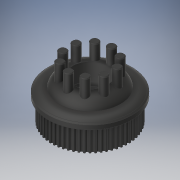
# Autodesk Inventor part: Orangatang Kegel Flat Face Adapter_2
Saved by Autodesk Inventor 2019.2 (Build 232265000, 265)
## iProperties
Created: 2018-11-27
Part Number: Orangatang Kegel Flat Face Adapter_2
Material: Aluminum 6061-AHC
Document SubType Name: Modeling
Designer: Petar
Density: 2.7 g/cm^3
Appearance: Smooth - Black
Author: Petar
Autodesk Inventor part; units mm, degrees
ref_plane "YZ Plane" through (0, 0, 0) normal (1, 0, 0) x (0, 1, 0)
ref_plane "XZ Plane" through (0, 0, 0) normal (0, 1, 0) x (-1, 0, 0)
ref_plane "XY Plane" through (0, 0, 0) normal (0, 0, 1) x (1, 0, 0)
derived "gates_P60-3M-09AL.ipt"
sketch "Sketch2_1" plane through (-27.813, -17.4625, 4.73202) normal (0, -1, 0) x (0.7504539, 0, 0.6609228)
  arc A0 (-0.667833, -0.547543) -> (0.667833, -0.547543) centre (0, 0) ccw
  arc A1 (-0.667833, -0.547543) -> (-1.061506, -0.54856) centre (-0.864255, -0.708586) ccw
  arc A2 (-1.061506, -0.54856) -> (-1.467465, -1.060953) centre (20.892519, -18.359372) ccw
  arc A3 (-1.467465, -1.060953) -> (-1.389566, -1.459114) centre (-1.254213, -1.225932) ccw
  arc A4 (-1.083217, -2.759174) -> (-1.389566, -1.459114) centre (-1.850942, -2.253958) ccw
  arc A5 (-2.411566, -2.898789) -> (-1.083217, -2.759174) centre (-1.804626, -2.284437) ccw
  arc A6 (-2.411566, -2.898789) -> (-2.802976, -2.94095) centre (-2.590078, -3.079481) ccw
  arc A7 (-2.802976, -2.94095) -> (-3.153152, -3.49297) centre (20.892519, -18.359372) ccw
  arc A8 (-3.153152, -3.49297) -> (-3.03406, -3.880808) centre (-2.923823, -3.634754) ccw
  arc A9 (-2.593496, -5.141723) -> (-3.03406, -3.880808) centre (-3.409825, -4.719524) ccw
  arc A10 (-3.899975, -5.419424) -> (-2.593496, -5.141723) centre (-3.360576, -4.744995) ccw
  arc A11 (-3.899975, -5.419424) -> (-4.284833, -5.502268) centre (-4.058622, -5.617785) ccw
  arc A12 (-4.284833, -5.502268) -> (-4.575389, -6.087867) centre (20.892519, -18.359372) ccw
  arc A13 (-4.575389, -6.087867) -> (-4.41641, -6.461132) centre (-4.332496, -6.204903) ccw
  arc A14 (-3.846458, -7.669088) -> (-4.41641, -6.461132) centre (-4.702447, -7.334531) ccw
  arc A15 (-5.116752, -8.081832) -> (-3.846458, -7.669088) centre (-4.650805, -7.354715) ccw
  arc A16 (-5.116752, -8.081832) -> (-5.490843, -8.20445) centre (-5.253795, -8.295689) ccw
  arc A17 (-5.490843, -8.20445) -> (-5.718595, -8.817212) centre (20.892519, -18.359372) ccw
  arc A18 (-5.718595, -8.817212) -> (-5.52147, -9.171815) centre (-5.464799, -8.908218) ccw
  arc A19 (-4.828374, -10.313578) -> (-5.52147, -9.171815) centre (-5.714644, -10.070329) ccw
  arc A20 (-6.048566, -10.856842) -> (-4.828374, -10.313578) centre (-5.661176, -10.085004) ccw
  arc A21 (-6.048566, -10.856842) -> (-6.40779, -11.017892) centre (-6.162504, -11.083853) ccw
  arc A22 (-6.40779, -11.017892) -> (-6.570244, -11.651104) centre (20.892519, -18.359372) ccw
  arc A23 (-6.570244, -11.651104) -> (-6.337133, -11.983159) centre (-6.308325, -11.715083) ccw
  arc A24 (-5.528487, -13.046219) -> (-6.337133, -11.983159) centre (-6.435328, -12.896943) ccw
  arc A25 (-6.685208, -13.714052) -> (-5.528487, -13.046219) centre (-6.380619, -12.905949) ccw
  arc A26 (-6.685208, -13.714052) -> (-7.02563, -13.911769) centre (-6.774793, -13.951729) ccw
  arc A27 (-7.02563, -13.911769) -> (-7.121005, -14.558493) centre (20.892519, -18.359372) ccw
  arc A28 (-7.121005, -14.558493) -> (-6.854462, -14.864362) centre (-6.853833, -14.594743) ccw
  arc A29 (-5.939126, -15.837072) -> (-6.854462, -14.864362) centre (-6.856603, -15.783405) ccw
  arc A30 (-7.019703, -16.622157) -> (-5.939126, -15.837072) centre (-6.801252, -15.786643) ccw
  arc A31 (-7.019703, -16.622157) -> (-7.337593, -16.854375) centre (-7.083953, -16.867897) ccw
  arc A32 (-7.337593, -16.854375) -> (-7.364844, -17.507526) centre (20.892519, -18.359372) ccw
  arc A33 (-7.364844, -17.507526) -> (-7.067789, -17.783857) centre (-7.095347, -17.51565) ccw
  arc A34 (-6.055792, -18.65556) -> (-7.067789, -17.783857) centre (-6.973852, -18.698089) ccw
  arc A35 (-7.048385, -19.549295) -> (-6.055792, -18.65556) centre (-6.918466, -18.695524) ccw
  arc A36 (-7.048385, -19.549295) -> (-7.34026, -19.813469) centre (-7.086596, -19.800405) ccw
  arc A37 (-7.34026, -19.813469) -> (-7.29909, -20.465891) centre (20.892519, -18.359372) ccw
  arc A38 (-7.29909, -20.465891) -> (-6.974777, -20.709658) centre (-7.03022, -20.4458) ccw
  arc A39 (-5.877206, -21.470803) -> (-6.974777, -20.709658) centre (-6.785792, -21.609063) ccw
  arc A40 (-6.770941, -22.463397) -> (-5.877206, -21.470803) centre (-6.730978, -21.600722) ccw
  arc A41 (-6.770941, -22.463397) -> (-7.033604, -22.756633) centre (-6.782695, -22.717124) ccw
  arc A42 (-7.033604, -22.756633) -> (-6.924462, -23.401177) centre (20.892519, -18.359372) ccw
  arc A43 (-6.924462, -23.401177) -> (-6.576445, -23.609709) centre (-6.659165, -23.353092) ccw
  arc A44 (-5.405325, -24.251957) -> (-6.576445, -23.609709) centre (-6.294482, -24.484432) ccw
  arc A45 (-6.19041, -25.332533) -> (-5.405325, -24.251957) centre (-6.24084, -24.470407) ccw
  arc A46 (-6.19041, -25.332533) -> (-6.420982, -25.651619) centre (-6.175578, -25.5861) ccw
  arc A47 (-6.420982, -25.651619) -> (-6.245066, -26.281223) centre (20.892519, -18.359372) ccw
  arc A48 (-6.245066, -26.281223) -> (-5.877158, -26.452235) centre (-5.986248, -26.205671) ccw
  arc A49 (-4.64532, -26.96855) -> (-5.877158, -26.452235) centre (-5.505306, -27.292694) ccw
  arc A50 (-5.313153, -28.12527) -> (-4.64532, -26.96855) centre (-5.453423, -27.273138) ccw
  arc A51 (-5.313153, -28.12527) -> (-5.509109, -28.466709) centre (-5.271898, -28.375898) ccw
  arc A52 (-5.509109, -28.466709) -> (-5.268344, -29.074477) centre (20.892519, -18.359372) ccw
  arc A53 (-5.268344, -29.074477) -> (-4.884576, -29.206095) centre (-5.018842, -28.972284) ccw
  arc A54 (-3.605517, -29.590819) -> (-4.884576, -29.206095) centre (-4.426909, -30.00308) ccw
  arc A55 (-4.148782, -30.811011) -> (-3.605517, -29.590819) centre (-4.377355, -29.978209) ccw
  arc A56 (-4.148782, -30.811011) -> (-4.307974, -31.171062) centre (-4.081554, -31.055952) ccw
  arc A57 (-4.307974, -31.171062) -> (-4.004999, -31.750333) centre (20.892519, -18.359372) ccw
  arc A58 (-4.004999, -31.750333) -> (-3.609575, -31.841116) centre (-3.767545, -31.62262) ccw
  arc A59 (-2.297309, -32.090034) -> (-3.609575, -31.841116) centre (-3.071108, -32.585895) ccw
  arc A60 (-2.710052, -33.360328) -> (-2.297309, -32.090034) centre (-3.024425, -32.555981) ccw
  arc A61 (-2.710052, -33.360328) -> (-2.830737, -33.735047) centre (-2.61759, -33.596901) ccw
  arc A62 (-2.830737, -33.735047) -> (-2.468871, -34.279475) centre (20.892519, -18.359372) ccw
  arc A63 (-2.468871, -34.279475) -> (-2.066125, -34.328427) centre (-2.246068, -34.127641) ccw
  arc A64 (-0.735027, -34.438813) -> (-2.066125, -34.328427) centre (-1.452756, -35.012842) ccw
  arc A65 (-1.012728, -35.745291) -> (-0.735027, -34.438813) centre (-1.409456, -34.978211) ccw
  arc A66 (-1.012728, -35.745291) -> (-1.093582, -36.130573) centre (-0.896043, -35.970903) ccw
  arc A67 (-1.093582, -36.130573) -> (-0.676791, -36.634193) centre (20.892519, -18.359372) ccw
  arc A68 (-0.676791, -36.634193) -> (-0.271134, -36.640779) centre (-0.471079, -36.459902) ccw
  arc A69 (1.06421, -36.611422) -> (-0.271134, -36.640779) centre (0.410415, -37.25733) ccw
  arc A70 (0.924595, -37.939771) -> (1.06421, -36.611422) centre (0.449858, -37.218363) ccw
  arc A71 (0.924595, -37.939771) -> (0.884456, -38.331394) centre (1.064223, -38.15195) ccw
  arc A72 (0.884456, -38.331394) -> (1.351607, -38.788689) centre (20.892519, -18.359372) ccw
  arc A73 (1.351607, -38.788689) -> (1.75573, -38.752836) centre (1.537973, -38.593849) ccw
  arc A74 (3.08069, -38.584058) -> (1.75573, -38.752836) centre (2.497993, -39.294768) ccw
  arc A75 (3.08069, -39.919724) -> (3.08069, -38.584058) centre (2.533146, -39.251891) ccw
  arc A76 (3.08069, -39.919724) -> (3.081707, -40.313397) centre (3.241732, -40.116146) ccw
  arc A77 (3.081707, -40.313397) -> (3.594099, -40.719356) centre (20.892519, -18.359372) ccw
  arc A78 (3.594099, -40.719356) -> (3.992261, -40.641457) centre (3.759078, -40.506104) ccw
  arc A79 (5.29232, -40.335108) -> (3.992261, -40.641457) centre (4.787105, -41.102833) ccw
  arc A80 (5.431935, -41.663458) -> (5.29232, -40.335108) centre (4.817584, -41.056517) ccw
  arc A81 (5.431935, -41.663458) -> (5.474097, -42.054867) centre (5.612627, -41.84197) ccw
  arc A82 (5.474097, -42.054867) -> (6.026116, -42.405043) centre (20.892519, -18.359372) ccw
  arc A83 (6.026116, -42.405043) -> (6.413954, -42.285952) centre (6.167901, -42.175714) ccw
  arc A84 (7.67487, -41.845388) -> (6.413954, -42.285952) centre (7.252671, -42.661716) ccw
  arc A85 (7.95257, -43.151866) -> (7.67487, -41.845388) centre (7.278142, -42.612468) ccw
  arc A86 (7.95257, -43.151866) -> (8.035414, -43.536725) centre (8.150932, -43.310513) ccw
  arc A87 (8.035414, -43.536725) -> (8.621013, -43.827281) centre (20.892519, -18.359372) ccw
  arc A88 (8.621013, -43.827281) -> (8.994278, -43.668301) centre (8.738049, -43.584387) ccw
  arc A89 (10.202235, -43.098349) -> (8.994278, -43.668301) centre (9.867678, -43.954338) ccw
  arc A90 (10.614978, -44.368643) -> (10.202235, -43.098349) centre (9.887862, -43.902697) ccw
  arc A91 (10.614978, -44.368643) -> (10.737597, -44.742734) centre (10.828836, -44.505687) ccw
  arc A92 (10.737597, -44.742734) -> (11.350359, -44.970486) centre (20.892519, -18.359372) ccw
  arc A93 (11.350359, -44.970486) -> (11.704961, -44.773361) centre (11.441365, -44.71669) ccw
  arc A94 (12.846724, -44.080266) -> (11.704961, -44.773361) centre (12.603476, -44.966536) ccw
  arc A95 (13.389989, -45.300457) -> (12.846724, -44.080266) centre (12.618151, -44.913068) ccw
  arc A96 (13.389989, -45.300457) -> (13.551039, -45.659681) centre (13.617, -45.414396) ccw
  arc A97 (13.551039, -45.659681) -> (14.184251, -45.822135) centre (20.892519, -18.359372) ccw
  arc A98 (14.184251, -45.822135) -> (14.516305, -45.589024) centre (14.248229, -45.560216) ccw
  arc A99 (15.579365, -44.780378) -> (14.516305, -45.589024) centre (15.43009, -45.68722) ccw
  arc A100 (16.247199, -45.937099) -> (15.579365, -44.780378) centre (15.439095, -45.632511) ccw
  arc A101 (16.247199, -45.937099) -> (16.444915, -46.277521) centre (16.484876, -46.026684) ccw
  arc A102 (16.444915, -46.277521) -> (17.09164, -46.372896) centre (20.892519, -18.359372) ccw
  arc A103 (17.09164, -46.372896) -> (17.397509, -46.106353) centre (17.12789, -46.105725) ccw
  arc A104 (18.370219, -45.191017) -> (17.397509, -46.106353) centre (18.316551, -46.108494) ccw
  arc A105 (19.155304, -46.271594) -> (18.370219, -45.191017) centre (18.319789, -46.053144) ccw
  arc A106 (19.155304, -46.271594) -> (19.387521, -46.589484) centre (19.401043, -46.335844) ccw
  arc A107 (19.387521, -46.589484) -> (20.040672, -46.616735) centre (20.892519, -18.359372) ccw
  arc A108 (20.040672, -46.616735) -> (20.317004, -46.31968) centre (20.048796, -46.347238) ccw
  arc A109 (21.188707, -45.307683) -> (20.317004, -46.31968) centre (21.231236, -46.225744) ccw
  arc A110 (22.082442, -46.300276) -> (21.188707, -45.307683) centre (21.22867, -46.170358) ccw
  arc A111 (22.082442, -46.300276) -> (22.346616, -46.592151) centre (22.333551, -46.338488) ccw
  arc A112 (22.346616, -46.592151) -> (22.999037, -46.550981) centre (20.892519, -18.359372) ccw
  arc A113 (22.999037, -46.550981) -> (23.242805, -46.226668) centre (22.978947, -46.282111) ccw
  arc A114 (24.00395, -45.129097) -> (23.242805, -46.226668) centre (24.142209, -46.037683) ccw
  arc A115 (24.996543, -46.022832) -> (24.00395, -45.129097) centre (24.133868, -45.982869) ccw
  arc A116 (24.996543, -46.022832) -> (25.289779, -46.285495) centre (25.250271, -46.034586) ccw
  arc A117 (25.289779, -46.285495) -> (25.934323, -46.176353) centre (20.892519, -18.359372) ccw
  arc A118 (25.934323, -46.176353) -> (26.142855, -45.828337) centre (25.886238, -45.911056) ccw
  arc A119 (26.785103, -44.657217) -> (26.142855, -45.828337) centre (27.017578, -45.546373) ccw
  arc A120 (27.86568, -45.442302) -> (26.785103, -44.657217) centre (27.003553, -45.492731) ccw
  arc A121 (27.86568, -45.442302) -> (28.184765, -45.672874) centre (28.119246, -45.427469) ccw
  arc A122 (28.184765, -45.672874) -> (28.81437, -45.496957) centre (20.892519, -18.359372) ccw
  arc A123 (28.81437, -45.496957) -> (28.985382, -45.129049) centre (28.738817, -45.238139) ccw
  arc A124 (29.501696, -43.897212) -> (28.985382, -45.129049) centre (29.82584, -44.757197) ccw
  arc A125 (30.658417, -44.565045) -> (29.501696, -43.897212) centre (29.806285, -44.705315) ccw
  arc A126 (30.658417, -44.565045) -> (30.999856, -44.761) centre (30.909044, -44.523789) ccw
  arc A127 (30.999856, -44.761) -> (31.607623, -44.520235) centre (20.892519, -18.359372) ccw
  arc A128 (31.607623, -44.520235) -> (31.739241, -44.136468) centre (31.505431, -44.270733) ccw
  arc A129 (32.123965, -42.857409) -> (31.739241, -44.136468) centre (32.536226, -43.678801) ccw
  arc A130 (33.344157, -43.400673) -> (32.123965, -42.857409) centre (32.511355, -43.629247) ccw
  arc A131 (33.344157, -43.400673) -> (33.704208, -43.559865) centre (33.589099, -43.333445) ccw
  arc A132 (33.704208, -43.559865) -> (34.283479, -43.25689) centre (20.892519, -18.359372) ccw
  arc A133 (34.283479, -43.25689) -> (34.374262, -42.861467) centre (34.155767, -43.019436) ccw
  arc A134 (34.62318, -41.5492) -> (34.374262, -42.861467) centre (35.119042, -42.322999) ccw
  arc A135 (35.893474, -41.961943) -> (34.62318, -41.5492) centre (35.089127, -42.276316) ccw
  arc A136 (35.893474, -41.961943) -> (36.268193, -42.082628) centre (36.130047, -41.869481) ccw
  arc A137 (36.268193, -42.082628) -> (36.812622, -41.720762) centre (20.892519, -18.359372) ccw
  arc A138 (36.812622, -41.720762) -> (36.861574, -41.318016) centre (36.660788, -41.497959) ccw
  arc A139 (36.971959, -39.986919) -> (36.861574, -41.318016) centre (37.545989, -40.704647) ccw
  arc A140 (38.278438, -40.264619) -> (36.971959, -39.986919) centre (37.511358, -40.661347) ccw
  arc A141 (38.278438, -40.264619) -> (38.663719, -40.345474) centre (38.50405, -40.147935) ccw
  arc A142 (38.663719, -40.345474) -> (39.16734, -39.928682) centre (20.892519, -18.359372) ccw
  arc A143 (39.16734, -39.928682) -> (39.173925, -39.523025) centre (38.993048, -39.722971) ccw
  arc A144 (39.144569, -38.187682) -> (39.173925, -39.523025) centre (39.790476, -38.841476) ccw
  arc A145 (40.472918, -38.327297) -> (39.144569, -38.187682) centre (39.751509, -38.802033) ccw
  arc A146 (40.472918, -38.327297) -> (40.86454, -38.367435) centre (40.685097, -38.187668) ccw
  arc A147 (40.86454, -38.367435) -> (41.321835, -37.900284) centre (20.892519, -18.359372) ccw
  arc A148 (41.321835, -37.900284) -> (41.285982, -37.496161) centre (41.126996, -37.713918) ccw
  arc A149 (41.117205, -36.171201) -> (41.285982, -37.496161) centre (41.827914, -36.753898) ccw
  arc A150 (42.452871, -36.171201) -> (41.117205, -36.171201) centre (41.785038, -36.718745) ccw
  arc A151 (42.452871, -36.171201) -> (42.846543, -36.170184) centre (42.649292, -36.010159) ccw
  arc A152 (42.846543, -36.170184) -> (43.252503, -35.657792) centre (20.892519, -18.359372) ccw
  arc A153 (43.252503, -35.657792) -> (43.174604, -35.25963) centre (43.03925, -35.492813) ccw
  arc A154 (42.868255, -33.959571) -> (43.174604, -35.25963) centre (43.63598, -34.464787) ccw
  arc A155 (44.196604, -33.819956) -> (42.868255, -33.959571) centre (43.589663, -34.434307) ccw
  arc A156 (44.196604, -33.819956) -> (44.588014, -33.777794) centre (44.375116, -33.639264) ccw
  arc A157 (44.588014, -33.777794) -> (44.93819, -33.225775) centre (20.892519, -18.359372) ccw
  arc A158 (44.93819, -33.225775) -> (44.819098, -32.837937) centre (44.70886, -33.08399) ccw
  arc A159 (44.378534, -31.577021) -> (44.819098, -32.837937) centre (45.194863, -31.99922) ccw
  arc A160 (45.685013, -31.299321) -> (44.378534, -31.577021) centre (45.145614, -31.973749) ccw
  arc A161 (45.685013, -31.299321) -> (46.069871, -31.216477) centre (45.84366, -31.100959) ccw
  arc A162 (46.069871, -31.216477) -> (46.360427, -30.630878) centre (20.892519, -18.359372) ccw
  arc A163 (46.360427, -30.630878) -> (46.201448, -30.257613) centre (46.117534, -30.513842) ccw
  arc A164 (45.631496, -29.049657) -> (46.201448, -30.257613) centre (46.487484, -29.384213) ccw
  arc A165 (46.90179, -28.636913) -> (45.631496, -29.049657) centre (46.435843, -29.36403) ccw
  arc A166 (46.90179, -28.636913) -> (47.27588, -28.514295) centre (47.038833, -28.423055) ccw
  arc A167 (47.27588, -28.514295) -> (47.503633, -27.901532) centre (20.892519, -18.359372) ccw
  arc A168 (47.503633, -27.901532) -> (47.306508, -27.54693) centre (47.249836, -27.810526) ccw
  arc A169 (46.613412, -26.405167) -> (47.306508, -27.54693) centre (47.499682, -26.648416) ccw
  arc A170 (47.833604, -25.861903) -> (46.613412, -26.405167) centre (47.446214, -26.633741) ccw
  arc A171 (47.833604, -25.861903) -> (48.192828, -25.700853) centre (47.947542, -25.634891) ccw
  arc A172 (48.192828, -25.700853) -> (48.355282, -25.06764) centre (20.892519, -18.359372) ccw
  arc A173 (48.355282, -25.06764) -> (48.12217, -24.735586) centre (48.093363, -25.003662) ccw
  arc A174 (47.313525, -23.672526) -> (48.12217, -24.735586) centre (48.220366, -23.821802) ccw
  arc A175 (48.470246, -23.004693) -> (47.313525, -23.672526) centre (48.165657, -23.812796) ccw
  arc A176 (48.470246, -23.004693) -> (48.810668, -22.806976) centre (48.559831, -22.767015) ccw
  arc A177 (48.810668, -22.806976) -> (48.906043, -22.160251) centre (20.892519, -18.359372) ccw
  arc A178 (48.906043, -22.160251) -> (48.639499, -21.854383) centre (48.638871, -22.124002) ccw
  arc A179 (47.724164, -20.881673) -> (48.639499, -21.854383) centre (48.641641, -20.93534) ccw
  arc A180 (48.80474, -20.096588) -> (47.724164, -20.881673) centre (48.58629, -20.932102) ccw
  arc A181 (48.80474, -20.096588) -> (49.12263, -19.86437) centre (48.86899, -19.850848) ccw
  arc A182 (49.12263, -19.86437) -> (49.149882, -19.211219) centre (20.892519, -18.359372) ccw
  arc A183 (49.149882, -19.211219) -> (48.852827, -18.934887) centre (48.880385, -19.203095) ccw
  arc A184 (47.840829, -18.063185) -> (48.852827, -18.934887) centre (48.75889, -18.020655) ccw
  arc A185 (48.833423, -17.169449) -> (47.840829, -18.063185) centre (48.703504, -18.023221) ccw
  arc A186 (48.833423, -17.169449) -> (49.125298, -16.905275) centre (48.871634, -16.91834) ccw
  arc A187 (49.125298, -16.905275) -> (49.084127, -16.252854) centre (20.892519, -18.359372) ccw
  arc A188 (49.084127, -16.252854) -> (48.759815, -16.009087) centre (48.815257, -16.272944) ccw
  arc A189 (47.662244, -15.247942) -> (48.759815, -16.009087) centre (48.57083, -15.109682) ccw
  arc A190 (48.555979, -14.255348) -> (47.662244, -15.247942) centre (48.516015, -15.118023) ccw
  arc A191 (48.555979, -14.255348) -> (48.818641, -13.962112) centre (48.567733, -14.00162) ccw
  arc A192 (48.818641, -13.962112) -> (48.7095, -13.317568) centre (20.892519, -18.359372) ccw
  arc A193 (48.7095, -13.317568) -> (48.361483, -13.109036) centre (48.444202, -13.365653) ccw
  arc A194 (47.190363, -12.466788) -> (48.361483, -13.109036) centre (48.07952, -12.234313) ccw
  arc A195 (47.975448, -11.386212) -> (47.190363, -12.466788) centre (48.025878, -12.248338) ccw
  arc A196 (47.975448, -11.386212) -> (48.20602, -11.067126) centre (47.960616, -11.132645) ccw
  arc A197 (48.20602, -11.067126) -> (48.030103, -10.437521) centre (20.892519, -18.359372) ccw
  arc A198 (48.030103, -10.437521) -> (47.662196, -10.266509) centre (47.771286, -10.513074) ccw
  arc A199 (46.430358, -9.750195) -> (47.662196, -10.266509) centre (47.290343, -9.426051) ccw
  arc A200 (47.098191, -8.593474) -> (46.430358, -9.750195) centre (47.238461, -9.445606) ccw
  arc A201 (47.098191, -8.593474) -> (47.294147, -8.252036) centre (47.056935, -8.342847) ccw
  arc A202 (47.294147, -8.252036) -> (47.053382, -7.644268) centre (20.892519, -18.359372) ccw
  arc A203 (47.053382, -7.644268) -> (46.669614, -7.51265) centre (46.803879, -7.746461) ccw
  arc A204 (45.390555, -7.127926) -> (46.669614, -7.51265) centre (46.211947, -6.715665) ccw
  arc A205 (45.933819, -5.907734) -> (45.390555, -7.127926) centre (46.162393, -6.740536) ccw
  arc A206 (45.933819, -5.907734) -> (46.093011, -5.547683) centre (45.866592, -5.662793) ccw
  arc A207 (46.093011, -5.547683) -> (45.790037, -4.968412) centre (20.892519, -18.359372) ccw
  arc A208 (45.790037, -4.968412) -> (45.394613, -4.877629) centre (45.552583, -5.096125) ccw
  arc A209 (44.082346, -4.628711) -> (45.394613, -4.877629) centre (44.856146, -4.132849) ccw
  arc A210 (44.49509, -3.358417) -> (44.082346, -4.628711) centre (44.809463, -4.162764) ccw
  arc A211 (44.49509, -3.358417) -> (44.615774, -2.983698) centre (44.402627, -3.121844) ccw
  arc A212 (44.615774, -2.983698) -> (44.253909, -2.43927) centre (20.892519, -18.359372) ccw
  arc A213 (44.253909, -2.43927) -> (43.851162, -2.390317) centre (44.031106, -2.591104) ccw
  arc A214 (42.520065, -2.279932) -> (43.851162, -2.390317) centre (43.237794, -1.705903) ccw
  arc A215 (42.797766, -0.973453) -> (42.520065, -2.279932) centre (43.194494, -1.740533) ccw
  arc A216 (42.797766, -0.973453) -> (42.87862, -0.588172) centre (42.681081, -0.747841) ccw
  arc A217 (42.87862, -0.588172) -> (42.461829, -0.084552) centre (20.892519, -18.359372) ccw
  arc A218 (42.461829, -0.084552) -> (42.056172, -0.077966) centre (42.256117, -0.258843) ccw
  arc A219 (40.720828, -0.107323) -> (42.056172, -0.077966) centre (41.374622, 0.538585) ccw
  arc A220 (40.860443, 1.221027) -> (40.720828, -0.107323) centre (41.33518, 0.499618) ccw
  arc A221 (40.860443, 1.221027) -> (40.900582, 1.612649) centre (40.720815, 1.433206) ccw
  arc A222 (40.900582, 1.612649) -> (40.433431, 2.069944) centre (20.892519, -18.359372) ccw
  arc A223 (40.433431, 2.069944) -> (40.029308, 2.034091) centre (40.247065, 1.875105) ccw
  arc A224 (38.704348, 1.865313) -> (40.029308, 2.034091) centre (39.287045, 2.576023) ccw
  arc A225 (38.704348, 3.20098) -> (38.704348, 1.865313) centre (39.251891, 2.533146) ccw
  arc A226 (38.704348, 3.20098) -> (38.703331, 3.594652) centre (38.543306, 3.397401) ccw
  arc A227 (38.703331, 3.594652) -> (38.190939, 4.000612) centre (20.892519, -18.359372) ccw
  arc A228 (38.190939, 4.000612) -> (37.792777, 3.922712) centre (38.02596, 3.787359) ccw
  arc A229 (36.492717, 3.616364) -> (37.792777, 3.922712) centre (36.997933, 4.384088) ccw
  arc A230 (36.353102, 4.944713) -> (36.492717, 3.616364) centre (36.967454, 4.337772) ccw
  arc A231 (36.353102, 4.944713) -> (36.310941, 5.336122) centre (36.172411, 5.123225) ccw
  arc A232 (36.310941, 5.336122) -> (35.758921, 5.686298) centre (20.892519, -18.359372) ccw
  arc A233 (35.758921, 5.686298) -> (35.371083, 5.567207) centre (35.617137, 5.456969) ccw
  arc A234 (34.110168, 5.126643) -> (35.371083, 5.567207) centre (34.532367, 5.942971) ccw
  arc A235 (33.832467, 6.433122) -> (34.110168, 5.126643) centre (34.506896, 5.893723) ccw
  arc A236 (33.832467, 6.433122) -> (33.749623, 6.81798) centre (33.634106, 6.591768) ccw
  arc A237 (33.749623, 6.81798) -> (33.164025, 7.108536) centre (20.892519, -18.359372) ccw
  arc A238 (33.164025, 7.108536) -> (32.79076, 6.949557) centre (33.046988, 6.865642) ccw
  arc A239 (31.582803, 6.379605) -> (32.79076, 6.949557) centre (31.91736, 7.235593) ccw
  arc A240 (31.17006, 7.649899) -> (31.582803, 6.379605) centre (31.897176, 7.183952) ccw
  arc A241 (31.17006, 7.649899) -> (31.047441, 8.023989) centre (30.956202, 7.786942) ccw
  arc A242 (31.047441, 8.023989) -> (30.434679, 8.251742) centre (20.892519, -18.359372) ccw
  arc A243 (30.434679, 8.251742) -> (30.080076, 8.054617) centre (30.343673, 7.997945) ccw
  arc A244 (28.938313, 7.361521) -> (30.080076, 8.054617) centre (29.181562, 8.247791) ccw
  arc A245 (28.395049, 8.581713) -> (28.938313, 7.361521) centre (29.166887, 8.194323) ccw
  arc A246 (28.395049, 8.581713) -> (28.233999, 8.940937) centre (28.168038, 8.695651) ccw
  arc A247 (28.233999, 8.940937) -> (27.600787, 9.103391) centre (20.892519, -18.359372) ccw
  arc A248 (27.600787, 9.103391) -> (27.268732, 8.870279) centre (27.536809, 8.841472) ccw
  arc A249 (26.205672, 8.061634) -> (27.268732, 8.870279) centre (26.354948, 8.968475) ccw
  arc A250 (25.537839, 9.218355) -> (26.205672, 8.061634) centre (26.345942, 8.913766) ccw
  arc A251 (25.537839, 9.218355) -> (25.340122, 9.558776) centre (25.300162, 9.30794) ccw
  arc A252 (25.340122, 9.558776) -> (24.693398, 9.654152) centre (20.892519, -18.359372) ccw
  arc A253 (24.693398, 9.654152) -> (24.387529, 9.387608) centre (24.657148, 9.38698) ccw
  arc A254 (23.414819, 8.472272) -> (24.387529, 9.387608) centre (23.468486, 9.389749) ccw
  arc A255 (22.629734, 9.552849) -> (23.414819, 8.472272) centre (23.465249, 9.334399) ccw
  arc A256 (22.629734, 9.552849) -> (22.397517, 9.870739) centre (22.383995, 9.617099) ccw
  arc A257 (22.397517, 9.870739) -> (21.744366, 9.897991) centre (20.892519, -18.359372) ccw
  arc A258 (21.744366, 9.897991) -> (21.468034, 9.600935) centre (21.736241, 9.628493) ccw
  arc A259 (20.596331, 8.588938) -> (21.468034, 9.600935) centre (20.553802, 9.506999) ccw
  arc A260 (19.702596, 9.581531) -> (20.596331, 8.588938) centre (20.556368, 9.451613) ccw
  arc A261 (19.702596, 9.581531) -> (19.438422, 9.873407) centre (19.451487, 9.619743) ccw
  arc A262 (19.438422, 9.873407) -> (18.786, 9.832236) centre (20.892519, -18.359372) ccw
  arc A263 (18.786, 9.832236) -> (18.542233, 9.507924) centre (18.806091, 9.563366) ccw
  arc A264 (17.781088, 8.410352) -> (18.542233, 9.507924) centre (17.642828, 9.318938) ccw
  arc A265 (16.788495, 9.304087) -> (17.781088, 8.410352) centre (17.65117, 9.264124) ccw
  arc A266 (16.788495, 9.304087) -> (16.495259, 9.56675) centre (16.534767, 9.315841) ccw
  arc A267 (16.495259, 9.56675) -> (15.850715, 9.457608) centre (20.892519, -18.359372) ccw
  arc A268 (15.850715, 9.457608) -> (15.642183, 9.109592) centre (15.8988, 9.192311) ccw
  arc A269 (14.999935, 7.938472) -> (15.642183, 9.109592) centre (14.767459, 8.827628) ccw
  arc A270 (13.919358, 8.723557) -> (14.999935, 7.938472) centre (14.781484, 8.773986) ccw
  arc A271 (13.919358, 8.723557) -> (13.600273, 8.954129) centre (13.665791, 8.708725) ccw
  arc A272 (13.600273, 8.954129) -> (12.970668, 8.778212) centre (20.892519, -18.359372) ccw
  arc A273 (12.970668, 8.778212) -> (12.799656, 8.410304) centre (13.046221, 8.519394) ccw
  arc A274 (12.283342, 7.178467) -> (12.799656, 8.410304) centre (11.959198, 8.038452) ccw
  arc A275 (11.126621, 7.8463) -> (12.283342, 7.178467) centre (11.978753, 7.98657) ccw
  arc A276 (11.126621, 7.8463) -> (10.785182, 8.042255) centre (10.875994, 7.805044) ccw
  arc A277 (10.785182, 8.042255) -> (10.177415, 7.801491) centre (20.892519, -18.359372) ccw
  arc A278 (10.177415, 7.801491) -> (10.045796, 7.417723) centre (10.279607, 7.551988) ccw
  arc A279 (9.661073, 6.138664) -> (10.045796, 7.417723) centre (9.248811, 6.960056) ccw
  arc A280 (8.440881, 6.681928) -> (9.661073, 6.138664) centre (9.273683, 6.910502) ccw
  arc A281 (8.440881, 6.681928) -> (8.080829, 6.84112) centre (8.195939, 6.614701) ccw
  arc A282 (8.080829, 6.84112) -> (7.501558, 6.538145) centre (20.892519, -18.359372) ccw
  arc A283 (7.501558, 6.538145) -> (7.410776, 6.142722) centre (7.629271, 6.300692) ccw
  arc A284 (7.161858, 4.830455) -> (7.410776, 6.142722) centre (6.665996, 5.604254) ccw
  arc A285 (5.891563, 5.243199) -> (7.161858, 4.830455) centre (6.695911, 5.557572) ccw
  arc A286 (5.891563, 5.243199) -> (5.516844, 5.363883) centre (5.654991, 5.150736) ccw
  arc A287 (5.516844, 5.363883) -> (4.972416, 5.002018) centre (20.892519, -18.359372) ccw
  arc A288 (4.972416, 5.002018) -> (4.923464, 4.599271) centre (5.12425, 4.779214) ccw
  arc A289 (4.813078, 3.268174) -> (4.923464, 4.599271) centre (4.239049, 3.985903) ccw
  arc A290 (3.5066, 3.545875) -> (4.813078, 3.268174) centre (4.27368, 3.942603) ccw
  arc A291 (3.5066, 3.545875) -> (3.121319, 3.626729) centre (3.280988, 3.42919) ccw
  arc A292 (3.121319, 3.626729) -> (2.617698, 3.209938) centre (20.892519, -18.359372) ccw
  arc A293 (2.617698, 3.209938) -> (2.611112, 2.80428) centre (2.791989, 3.004226) ccw
  arc A294 (2.640469, 1.468937) -> (2.611112, 2.80428) centre (1.994561, 2.122731) ccw
  arc A295 (1.31212, 1.608552) -> (2.640469, 1.468937) centre (2.033528, 2.083288) ccw
  arc A296 (1.31212, 1.608552) -> (0.920498, 1.648691) centre (1.099941, 1.468924) ccw
  arc A297 (0.920498, 1.648691) -> (0.463203, 1.18154) centre (20.892519, -18.359372) ccw
  arc A298 (0.463203, 1.18154) -> (0.499056, 0.777416) centre (0.658042, 0.995173) ccw
  arc A299 (0.667833, -0.547543) -> (0.499056, 0.777416) centre (-0.042877, 0.035154) ccw
  circle A300 centre (20.892519, -18.359372) radius 4.564063
  point P0 (17.744874, -21.933409)
sketch "Sketch1" plane through (0, 0, 0) normal (0, 1, 0) x (-1, 0, 0)
  circle A0 centre (0, 4.7625) radius 22.4
  circle A1 centre (0, 4.7625) radius 12.5
  circle A2 centre (0, 4.7625) radius 4.564063
  dimension "d0" = 44.8
  dimension "d1" = 25
  constraints: 3 coincident, 2 centre point
  measures "d0" diameter of A0
  measures "d1" diameter of A1
extrude "Extrusion1" add sketch "Sketch1" along normal blind 7 contours A0
fillet "Fillet1" radius 10 1 edges at (22.4, 7, 4.7625)
sketch "Sketch2" plane through (0, 0, 4.7625) normal (0, -1, 0) x (1, 0, 0)
  circle A0 centre (0, 0) radius 12.5 projected
  circle A1 centre (0, -15.85) radius 2.9
  dimension "d5" = 5.8
  dimension "d6" = 15.85
  constraints: 1 centre point
  measures "d5" diameter of A1
  measures "d6" distance of A0.centre A1.centre
extrude "Extrusion2" add sketch "Sketch2" against normal blind 18 contours A1
chamfer "Chamfer1" distance 0.5 angle 45 1 edges at (-2.9, 18, -11.0875)
pattern_circular "Circular Pattern1" count 10 over 360 about axis through (0, 0, 4.7625) along (0, 1, 0) of "Extrusion2", "Chamfer1"
ref_plane "Work Plane1" through (0, -20, 4.7625) normal (0, -1, 0) x (1, 0, 0)
sketch "Sketch3" plane through (0, -20, 4.7625) normal (0, -1, 0) x (1, 0, 0)
  arc A0 (0.469, -27.904741) -> (-0.469, -27.904741) centre (0, -27.904741) ccw
  line L0 (0, -4.7625) -> (0, -28.635741) construction
  circle A1 centre (0, -4.7625) radius 23.873241
  line L1 (0.469, -27.904741) -> (0.469, -28.631134)
  line L2 (-0.469, -27.904741) -> (-0.469, -28.631134)
  point P0 (0, -27.435741)
  dimension "d16" = 0.938
  dimension "d17" = 23.87324
  dimension "d50" = 1.2
  constraints: 6 end point, 6 point on circle, 2 centre point, 2 point on line, 2 tangent, 1 coincident, 1 parallel, 1 vertical
  measures "d16" diameter of A0
  measures "d17" distance of L0.start L0.end
  measures "d50" distance of point (0, -27.436) L0.end
sketch "Sketch4" plane through (0, 0, 4.7625) normal (0, -1, 0) x (1, 0, 0)
  circle A0 centre (0, 0) radius 12.5
  circle A1 centre (0, 0) radius 28.27
  circle A2 centre (0, 0) radius 30.67
  circle A3 centre (0, 0) radius 4.564063
  dimension "d18" = 2.4
  dimension "d53" = 56.54
  constraints: 2 centre point, 2 coincident
  measures "d18" radial gap between concentric circles of A1 A2
  measures "d53" diameter of A1
extrude "Extrusion3" add sketch "Sketch4" along normal blind 7 contours A1 | A2
chamfer "Chamfer2" distance 2.4 distance2 1 1 edges at (-30.67, -7, 4.7625) measured on face at (-30.17, -7, 4.7625)
extrude "Extrusion8" add sketch "Sketch2_1" against normal blind 11 and the other way blind 5
sketch "Sketch11" plane through (-27.813, -22.4625, 4.73202) normal (0, -1, 0) x (0.7504539, 0, 0.6609228)
  circle A0 centre (20.892519, -18.359372) radius 4.564062
  circle A1 centre (20.892519, -18.359372) radius 12.5
  point P0 (17.744874, -21.933409)
extrude "Extrusion9" cut sketch "Sketch11" against normal through all
chamfer "Chamfer5" distance 3 angle 45 1 edges at (-30.67, 0, 4.7625)
fillet "Fillet4" radius 7 1 edges at (-27.67, 0, 4.7625)
chamfer "Chamfer6" distance 9.5 distance2 14.65 1 edges at (-9.3807, -22.4625, -3.499) measured on face at (-9.7559, -22.4625, -3.8295)
fillet "Fillet5" radius 7 1 edges at (-9.3807, -7.8125, -3.499)
body "Solid1"
